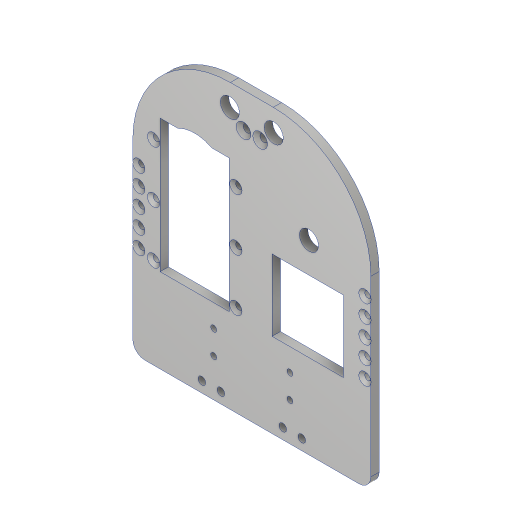
# Autodesk Inventor part: Box_Front
Saved by Autodesk Inventor 2023.2 (Build 272271000, 271)
## iProperties
Created: 2021-07-28
Part Number: Box_Front
Material: 알루미늄 6061
Document SubType Name: Modeling
Designer: user
Density: 2.7 g/cm^3
Appearance: 알루미늄 - 평지
Mass: 39.6776 g
Surface Area: 168.104 cm^2
Volume: 24.402 cm^3
Author: user
Autodesk Inventor part; units mm, degrees
ref_plane "YZ Plane" through (0, 0, 0) normal (1, 0, 0) x (0, 1, 0)
ref_plane "XZ Plane" through (0, 0, 0) normal (0, 1, 0) x (-1, 0, 0)
ref_plane "XY Plane" through (0, 0, 0) normal (0, 0, 1) x (1, 0, 0)
sketch "스케치1" plane through (0, 0, 0) normal (0, 0, 1) x (1, 0, 0)
  line L0 (-50.01, 54) -> (50.01, 54)
  line L1 (50.01, 54) -> (50.01, -40)
  line L2 (50.01, -40) -> (-50.01, -40)
  line L3 (-50.01, -40) -> (-50.01, 54)
  point P0 (0, 0)
  dimension "d0" = 100.02
  dimension "d1" = 50.01
  dimension "d2" = 94
  dimension "d40" = 40
  constraints: 8 end point, 2 parallel, 1 horizontal, 1 perpendicular
  measures "d0" distance of L1.end L2.end
  measures "d1" distance from line of L3 point (0, 0)
  measures "d2" distance between parallel lines of L2 L0
  measures "d40" distance from line of point (0, 0) L2
extrude "돌출1" add sketch "스케치1" along normal blind 3.5
sketch "스케치2" plane through (0, 0, 3.5) normal (0, 0, 1) x (1, 0, 0)
  circle A0 centre (-24.01, 13.1) radius 14
  line L0 (-50.01, -40) -> (50.01, -40) projected
  point P0 (0, 0)
  dimension "d6" = 28
  dimension "d7" = 24.01
  dimension "d8" = 53.1
  constraints: 1 centre point
  measures "d6" diameter of A0
  measures "d7" horizontal distance of point (0, 0) A0.centre
  measures "d8" distance from line of L0 A0.centre
extrude "돌출2" cut sketch "스케치2" against normal up to surface (3.5 mm away)
sketch "스케치3" plane through (0, 0, 3.5) normal (0, 0, 1) x (1, 0, 0)
  line L0 (-9.49, -29.6) -> (-38.53, -29.6)
  line L1 (-38.53, -29.6) -> (-38.53, 26.3)
  line L2 (-38.53, 26.3) -> (-9.49, 26.3)
  line L3 (-9.49, 26.3) -> (-9.49, -29.6)
  line L4 (-50.01, -40) -> (50.01, -40) projected
  circle A0 centre (-24.01, 13.1) radius 14 projected
  point P0 (0, 0)
  dimension "d11" = 10.4
  dimension "d12" = 55.9
  dimension "d13" = 29.04
  dimension "d14" = 14.52
  constraints: 8 end point, 2 parallel, 1 horizontal, 1 perpendicular
  measures "d11" distance between parallel lines of L4 L0
  measures "d12" distance between parallel lines of L0 L2
  measures "d13" distance between parallel lines of L3 L1
  measures "d14" distance from line of L1 A0.centre
extrude "돌출3" cut sketch "스케치3" against normal up to surface (3.5 mm away) contours L0 L1 L2 A0 L3 | A0 L2 picked at (-19.646, 17.031)
sketch "스케치4" plane through (0, 0, 3.5) normal (0, 0, 1) x (1, 0, 0)
  line L0 (-38.53, -29.6) -> (-38.53, 26.3) projected
  line L1 (-9.49, 26.3) -> (-9.49, -29.6) projected
  line L2 (-9.49, -29.6) -> (-38.53, -29.6) projected
  arc A0 (-19.3452, 26.3) -> (-28.6748, 26.3) centre (-24.01, 13.1) ccw projected
  arc A1 (-16.8854, 26.3) -> (-31.1346, 26.3) centre (-24.01, 13.1) ccw
  line L3 (-38.53, 26.3) -> (-28.6748, 26.3) projected
  line L4 (-19.3452, 26.3) -> (-9.49, 26.3) projected
  point P0 (0, 0)
  constraints: 2 point on circle, 2 point on line, 1 centre point, 1 coincident
extrude "돌출4" cut sketch "스케치4" against normal up to surface (3.5 mm away)
sketch "스케치5" plane through (0, 0, 3.5) normal (0, 0, 1) x (1, 0, 0)
  arc A0 (-16.8854, 26.3) -> (-31.1346, 26.3) centre (-24.01, 13.1) ccw projected
  circle A1 centre (-24.01, 13.1) radius 5
  circle A2 centre (-6.71, -4.9) radius 1.705
  circle A3 centre (-6.71, 17.1) radius 1.705
  circle A4 centre (-6.71, -26.9) radius 1.7
  circle A5 centre (-13.01, -32.2) radius 1.705
  circle A6 centre (-35.01, -32.2) radius 1.705
  circle A7 centre (-41.31, -26.9) radius 1.705
  circle A8 centre (-41.31, -4.9) radius 1.705
  circle A9 centre (-41.31, 17.1) radius 1.705
  circle A10 centre (-41.31, 17.1) radius 1.35
  circle A11 centre (-41.31, -4.9) radius 1.35
  circle A12 centre (-41.31, -26.9) radius 1.35
  circle A13 centre (-35.01, -32.2) radius 1.35
  circle A14 centre (-13.01, -32.2) radius 1.35
  circle A15 centre (-6.71, -26.9) radius 1.35
  circle A16 centre (-6.71, -4.9) radius 1.35
  circle A17 centre (-6.71, 17.1) radius 1.35
  point P0 (0, 0)
  dimension "d20" = 3.41
  dimension "d21" = 2.7
  dimension "d22" = 2.7
  dimension "d23" = 2.7
  dimension "d24" = 2.7
  dimension "d25" = 2.7
  dimension "d26" = 2.7
  dimension "d27" = 2.7
  dimension "d28" = 2.7
  constraints: 17 centre point, 8 coincident
  measures "d20" diameter of A9
  measures "d21" diameter of A10
  measures "d22" diameter of A11
  measures "d23" diameter of A12
  measures "d24" diameter of A13
  measures "d25" diameter of A14
  measures "d26" diameter of A15
  measures "d27" diameter of A16
  measures "d28" diameter of A17
extrude "돌출5" cut sketch "스케치5" against normal up to surface (3.5 mm away) contours A10 | A11 | A12 | A15 | A16 | A17
sketch "스케치6" plane through (0, 0, 3.5) normal (0, 0, 1) x (1, 0, 0)
  arc A0 (-16.8854, 26.3) -> (-31.1346, 26.3) centre (-24.01, 13.1) ccw projected
  line L0 (-24.01, 13.1) -> (24.01, 13.1)
  line L1 (-24.01, 13.1) -> (24.01, 13.1) construction
  circle A1 centre (24.01, 13.1) radius 4.025
  point P0 (0, 0)
  dimension "d31" = 48.02
  dimension "d32" = 0
  dimension "d33" = 8.05
  constraints: 4 end point, 2 horizontal, 1 centre point, 1 coincident, 1 collinear
  measures "d31" distance of L0.start L0.end
  measures "d32" distance between parallel lines of L0 L1
  measures "d33" diameter of A1
extrude "돌출6" cut sketch "스케치6" against normal up to surface (3.5 mm away)
chamfer "모따기1" distance 1.25 angle 45 6 edges at (-42.66, 17.1, 3.5) (-42.66, -4.9, 3.5) (-42.66, -26.9, 3.5) (-8.06, -26.9, 3.5) (-8.06, -4.9, 3.5) (-8.06, 17.1, 3.5)
sketch "스케치7" plane through (0, 0, 3.5) normal (0, 0, 1) x (1, 0, 0)
  circle A0 centre (24.01, 13.1) radius 4.025 projected
  arc A1 (-16.8854, 26.3) -> (-31.1346, 26.3) centre (-24.01, 13.1) ccw projected
  line L0 (24.01, 13.1) -> (9.2184, 44.8208)
  line L1 (24.01, 13.1) -> (59.01, 13.1) construction
  line L2 (-24.01, 13.1) -> (-9.2184, 44.8208)
  line L3 (-24.01, 13.1) -> (10.99, 13.1) construction
  circle A2 centre (9.2184, 44.8208) radius 4.025
  circle A3 centre (-9.2184, 44.8208) radius 4.025
  point P0 (0, 0)
  dimension "d41" = 35
  dimension "d42" = 115
  dimension "d43" = 35
  dimension "d44" = 65
  dimension "d45" = 8.05
  dimension "d46" = 8.05
  constraints: 8 end point, 2 centre point, 2 coincident, 2 equal length, 2 horizontal
  measures "d41" distance of L0.start L0.end
  measures "d42" angle of L1 L0
  measures "d43" distance of L2.start L2.end
  measures "d44" angle of L3 L2
  measures "d45" diameter of A2
  measures "d46" diameter of A3
extrude "돌출7" cut sketch "스케치7" against normal up to surface (3.5 mm away) contours A2 | A3
fillet "모깎기1" radius 41 2 edges at (50.01, 54, 1.75) (-50.01, 54, 1.75)
sketch "스케치8" plane through (0, 0, 3.5) normal (0, 0, 1) x (1, 0, 0)
  circle A0 centre (47.51, -25.5) radius 1.35
  circle A1 centre (47.51, 4.5) radius 1.35
  circle A2 centre (47.51, -18) radius 1.35
  circle A3 centre (47.51, -10.5) radius 1.35
  circle A4 centre (47.51, -3) radius 1.35
  line L0 (50.01, -40) -> (50.01, 13) projected
  line L1 (-50.01, -40) -> (50.01, -40) projected
  point P0 (0, 0)
  dimension "d50" = 2.7
  dimension "d51" = 2.7
  dimension "d52" = 2.7
  dimension "d53" = 2.7
  dimension "d54" = 2.7
  dimension "d55" = 2.5
  dimension "d56" = 2.5
  dimension "d57" = 2.5
  dimension "d58" = 2.5
  dimension "d59" = 2.5
  dimension "d60" = 14.5
  dimension "d61" = 44.5
  dimension "d62" = 22
  dimension "d63" = 29.5
  dimension "d64" = 37
  constraints: 5 centre point
  measures "d50" diameter of A0
  measures "d51" diameter of A1
  measures "d52" diameter of A2
  measures "d53" diameter of A3
  measures "d54" diameter of A4
  measures "d55" distance from line of L0 A0.centre
  measures "d56" distance from line of L0 A1.centre
  measures "d57" distance from line of L0 A2.centre
  measures "d58" distance from line of L0 A3.centre
  measures "d59" distance from line of L0 A4.centre
  measures "d60" distance from line of L1 A0.centre
  measures "d61" distance from line of L1 A1.centre
  measures "d62" distance from line of L1 A2.centre
  measures "d63" distance from line of L1 A3.centre
  measures "d64" distance from line of L1 A4.centre
extrude "돌출8" cut sketch "스케치8" against normal up to surface (3.5 mm away)
chamfer "모따기2" distance 1.25 angle 45 5 edges at (46.16, -25.5, 3.5) (46.16, -18, 3.5) (46.16, -10.5, 3.5) (46.16, -3, 3.5) (46.16, 4.5, 3.5)
sketch "스케치9" plane through (0, 0, 3.5) normal (0, 0, 1) x (1, 0, 0)
  line L0 (0, 0) -> (0, -40)
  line L1 (-50.01, -40) -> (50.01, -40) projected
  circle A0 centre (47.51, 4.5) radius 1.35 projected
  circle A1 centre (47.51, -3) radius 1.35 projected
  circle A2 centre (47.51, -10.5) radius 1.35 projected
  circle A3 centre (47.51, -18) radius 1.35 projected
  circle A4 centre (47.51, -25.5) radius 1.35 projected
  circle A5 centre (-47.51, 4.5) radius 1.35
  circle A6 centre (-47.51, -3) radius 1.35
  circle A7 centre (-47.51, -10.5) radius 1.35
  circle A8 centre (-47.51, -18) radius 1.35
  circle A9 centre (-47.51, -25.5) radius 1.35
  constraints: 5 centre point, 5 symmetric about line, 2 end point, 1 midpoint, 5 other
extrude "돌출9" cut sketch "스케치9" against normal up to surface (3.5 mm away) contours A5 | A6 | A7 | A8 | A9
chamfer "모따기3" distance 1.25 angle 45 5 edges at (-48.86, 4.5, 3.5) (-48.86, -3, 3.5) (-48.86, -10.5, 3.5) (-48.86, -18, 3.5) (-48.86, -25.5, 3.5)
sketch "스케치10" plane through (0, 0, 3.5) normal (0, 0, 1) x (1, 0, 0)
  line L0 (-50.01, -26.2141) -> (-50.01, -40) projected
  line L1 (-50.01, -40) -> (50.01, -40) projected
  line L2 (50.01, -40) -> (50.01, -26.2141) projected
  line L3 (-50.01, -40) -> (50.01, -40)
  line L4 (50.01, -40) -> (50.01, -65)
  line L5 (50.01, -65) -> (-50.01, -65)
  line L6 (-50.01, -65) -> (-50.01, -40)
  point P0 (0, 0)
  dimension "d75" = 25
  dimension "d76" = 100.02
  constraints: 8 end point, 2 parallel, 1 horizontal, 1 perpendicular
  measures "d75" distance of L3.end L4.end
  measures "d76" distance between parallel lines of L4 L6
extrude "돌출10" add sketch "스케치10" against normal up to surface (3.5 mm away)
sketch "스케치11" plane through (0, 0, 3.5) normal (0, 0, 1) x (1, 0, 0)
  line L0 (-25, -58) -> (25, -58)
  line L1 (25, -58) -> (25, -63)
  line L2 (25, -63) -> (-25, -63)
  line L3 (-25, -63) -> (-25, -58)
  line L4 (50.01, -65) -> (-50.01, -65) projected
  circle A0 centre (-21, -60.5) radius 1.6
  circle A1 centre (-13, -60.5) radius 1.6
  circle A2 centre (13, -60.5) radius 1.6
  circle A3 centre (21, -60.5) radius 1.6
  point P0 (0, 0)
  dimension "d79" = 50
  dimension "d80" = 5
  dimension "d81" = 25
  dimension "d82" = 7
  dimension "d83" = 3.2
  dimension "d84" = 3.2
  dimension "d85" = 3.2
  dimension "d86" = 3.2
  dimension "d87" = 4
  dimension "d88" = 2.5
  dimension "d89" = 2.5
  dimension "d90" = 12
  dimension "d91" = 2.5
  dimension "d92" = 2.5
  dimension "d93" = 4
  dimension "d94" = 12
  constraints: 8 end point, 4 centre point, 2 parallel, 1 horizontal, 1 perpendicular
  measures "d79" distance of L1.end L2.end
  measures "d80" distance of L0.end L1.end
  measures "d81" distance from line of L1 point (0, 0)
  measures "d82" distance between parallel lines of L4 L0
  measures "d83" diameter of A0
  measures "d84" diameter of A1
  measures "d85" diameter of A2
  measures "d86" diameter of A3
  measures "d87" distance from line of L3 A0.centre
  measures "d88" distance from line of L2 A1.centre
  measures "d89" distance from line of L2 A0.centre
  measures "d90" distance from line of A1.centre L3
  measures "d91" distance from line of L2 A2.centre
  measures "d92" distance from line of L2 A3.centre
  measures "d93" distance from line of L1 A3.centre
  measures "d94" distance from line of L1 A2.centre
extrude "돌출11" cut sketch "스케치11" against normal up to surface (3.5 mm away) contours A0 | A1 | A2 | A3
fillet "모깎기2" radius 5 2 edges at (50.01, -65, 1.75) (-50.01, -65, 1.75)
sketch "스케치13" plane through (0, 0, 0) normal (0, 0, -1) x (-1, 0, 0)
  line L0 (9.49, 26.3) -> (16.8854, 26.3) projected
  line L1 (7, 36.3) -> (-7, 36.3)
  line L2 (-7, 36.3) -> (-7, 42.3)
  line L3 (-7, 42.3) -> (7, 42.3)
  line L4 (7, 42.3) -> (7, 36.3)
  circle A0 centre (3.5, 39.3) radius 1.6
  circle A1 centre (-3.5, 39.3) radius 1.6
  point P0 (0, 0)
  dimension "d124" = 14
  dimension "d125" = 6
  dimension "d126" = 7
  dimension "d127" = 16
  dimension "d128" = 3.2
  dimension "d129" = 3.2
  dimension "d130" = 3.5
  dimension "d131" = 3.5
  dimension "d132" = 3
  dimension "d133" = 3
  constraints: 8 end point, 2 centre point, 2 parallel, 1 horizontal, 1 perpendicular
  measures "d124" distance of L2.end L3.end
  measures "d125" distance of L1.end L2.end
  measures "d126" distance from line of point (0, 0) L2
  measures "d127" distance between parallel lines of L3 L0
  measures "d128" diameter of A0
  measures "d129" diameter of A1
  measures "d130" distance from line of L4 A0.centre
  measures "d131" distance from line of L2 A1.centre
  measures "d132" distance from line of L3 A0.centre
  measures "d133" distance from line of L3 A1.centre
extrude "돌출13" cut sketch "스케치13" against normal up to surface (3.5 mm away) contours A0 | A1
chamfer "모따기5" distance 1.5 angle 45 2 edges at (5.1, 39.3, 3.5) (-1.9, 39.3, 3.5)
sketch "스케치17" plane through (0, 0, 3.5) normal (0, 0, 1) x (1, 0, 0)
  line L0 (-20, -31.5) -> (20, -31.5)
  line L1 (20, -31.5) -> (20, -56.5)
  line L2 (20, -56.5) -> (-20, -56.5)
  line L3 (-20, -56.5) -> (-20, -31.5)
  line L4 (-20, -31.5) -> (20, -56.5) construction
  line L5 (20, -31.5) -> (-20, -56.5) construction
  line L6 (45.01, -65) -> (-45.01, -65) projected
  point P0 (0, 0)
  point P1 (0, -44)
  point P2 (0, -65)
  dimension "d150" = 40
  dimension "d151" = 25
  dimension "d152" = 21
  constraints: 12 end point, 3 midpoint, 2 parallel, 1 horizontal, 1 perpendicular, 1 vertical alignment
  measures "d150" distance of L1.end L2.end
  measures "d151" distance of L0.end L1.end
  measures "d152" distance of point (0, -44) point (0, -65)
extrude "돌출17" add sketch "스케치17" along normal blind 26
sketch "스케치19" plane through (0, 0, 29.5) normal (0, 0, 1) x (1, 0, 0)
  line L0 (-20, -56.5) -> (20, -56.5) projected
  line L1 (20, -56.5) -> (20, -31.5) projected
  line L2 (20, -31.5) -> (-20, -31.5) projected
  line L3 (-20, -31.5) -> (-20, -56.5) projected
  circle A0 centre (-16, -39) radius 1.25
  circle A1 centre (-16, -49) radius 1.25
  line L4 (20, -31.5) -> (-20, -31.5) projected
  line L5 (0, -31.5) -> (0, -56.5)
  circle A2 centre (16, -39) radius 1.25
  circle A3 centre (16, -49) radius 1.25
  point P0 (0, 0)
  dimension "d155" = 10
  dimension "d156" = 2.5
  dimension "d157" = 4
  dimension "d158" = 7.5
  constraints: 4 centre point, 2 end point, 2 midpoint, 2 symmetric about line, 1 equal radius, 1 vertical alignment, 2 other
  measures "d155" distance of A0.centre A1.centre
  measures "d156" diameter of A0
  measures "d157" distance from line of L3 A0.centre
  measures "d158" distance from line of L0 A1.centre
extrude "돌출18" cut sketch "스케치19" against normal blind 26 contours A0 | A1 | A2 | A3
sketch "스케치20" plane through (0, 0, 29.5) normal (0, 0, 1) x (1, 0, 0)
  circle A0 centre (16, -39) radius 1.25 projected
  circle A1 centre (-16, -49) radius 1.25 projected
  circle A2 centre (16, -49) radius 1.25 projected
  circle A3 centre (-16, -39) radius 1.25 projected
  line L0 (-20, -56.5) -> (20, -56.5) projected
  line L1 (20, -56.5) -> (20, -31.5) projected
  line L2 (20, -31.5) -> (-20, -31.5) projected
  line L3 (-20, -31.5) -> (-20, -56.5) projected
  line L4 (-6, -36.5) -> (6, -36.5)
  line L5 (10, -40.5) -> (10, -47.5)
  line L6 (6, -51.5) -> (-6, -51.5)
  line L7 (-10, -47.5) -> (-10, -40.5)
  line L8 (-10, -36.5) -> (10, -51.5) construction
  line L9 (10, -36.5) -> (-10, -51.5) construction
  line L10 (-20, -56.5) -> (20, -56.5) projected
  arc A4 (-6, -36.5) -> (-10, -40.5) centre (-6, -40.5) ccw
  arc A5 (10, -40.5) -> (6, -36.5) centre (6, -40.5) ccw
  arc A6 (6, -51.5) -> (10, -47.5) centre (6, -47.5) ccw
  arc A7 (-10, -47.5) -> (-6, -51.5) centre (-6, -47.5) ccw
  point P0 (0, 0)
  point P1 (0, -44)
  point P2 (0, -56.5)
  point P3 (0, -56.5)
  point P4 (0, -51.5)
  dimension "d161" = 20
  dimension "d162" = 15
  dimension "d164" = 5
  dimension "d165" = 4
  constraints: 12 end point, 8 point on circle, 8 point on line, 8 tangent, 5 midpoint, 4 centre point, 3 equal radius, 2 parallel, 1 horizontal, 1 perpendicular
  measures "d161" distance of L8.end L9.end
  measures "d162" distance of L9.start L8.end
  measures "d164" distance of point (0, -56.5) point (0, -51.5)
  measures "d165" radius of A4
extrude "돌출19" cut sketch "스케치20" against normal blind 26 contours L4 A5 L5 A6 L6 A7 L7 A4
fillet "모깎기3" radius 4 4 edges at (-20, -31.5, 16.5) (-20, -56.5, 16.5) (20, -56.5, 16.5) (20, -31.5, 16.5)
sketch "스케치21" plane through (0, 0, 29.5) normal (0, 0, 1) x (1, 0, 0)
  arc A0 (6, -51.5) -> (10, -47.5) centre (6, -47.5) ccw projected
  line L0 (6, -51.5) -> (-6, -51.5) projected
  arc A1 (-10, -47.5) -> (-6, -51.5) centre (-6, -47.5) ccw projected
  line L1 (-10, -47.5) -> (-10, -40.5) projected
  arc A2 (-6, -36.5) -> (-10, -40.5) centre (-6, -40.5) ccw projected
  line L2 (-6, -36.5) -> (6, -36.5) projected
  arc A3 (10, -40.5) -> (6, -36.5) centre (6, -40.5) ccw projected
  line L3 (10, -40.5) -> (10, -47.5) projected
  circle A4 centre (16, -39) radius 1.25 projected
  circle A5 centre (-16, -49) radius 1.25 projected
  circle A6 centre (16, -49) radius 1.25 projected
  circle A7 centre (-16, -39) radius 1.25 projected
  arc A8 (20, -35.5) -> (16, -31.5) centre (16, -35.5) ccw projected
  line L4 (16, -31.5) -> (-16, -31.5) projected
  arc A9 (-16, -31.5) -> (-20, -35.5) centre (-16, -35.5) ccw projected
  line L5 (-20, -35.5) -> (-20, -52.5) projected
  arc A10 (-20, -52.5) -> (-16, -56.5) centre (-16, -52.5) ccw projected
  line L6 (-16, -56.5) -> (16, -56.5) projected
  arc A11 (16, -56.5) -> (20, -52.5) centre (16, -52.5) ccw projected
  line L7 (20, -52.5) -> (20, -35.5) projected
  point P0 (0, 0)
extrude "돌출20" cut sketch "스케치21" against normal up to surface (29.5 mm away) contours A4 | A5 | A6 | A7
sketch "스케치22" plane through (0, 0, 29.5) normal (0, 0, 1) x (1, 0, 0)
  arc A0 (6, -51.5) -> (10, -47.5) centre (6, -47.5) ccw projected
  line L0 (6, -51.5) -> (-6, -51.5) projected
  arc A1 (-10, -47.5) -> (-6, -51.5) centre (-6, -47.5) ccw projected
  line L1 (-10, -47.5) -> (-10, -40.5) projected
  arc A2 (-6, -36.5) -> (-10, -40.5) centre (-6, -40.5) ccw projected
  line L2 (-6, -36.5) -> (6, -36.5) projected
  arc A3 (10, -40.5) -> (6, -36.5) centre (6, -40.5) ccw projected
  line L3 (10, -40.5) -> (10, -47.5) projected
  circle A4 centre (16, -39) radius 1.25 projected
  circle A5 centre (-16, -49) radius 1.25 projected
  circle A6 centre (16, -49) radius 1.25 projected
  circle A7 centre (-16, -39) radius 1.25 projected
  arc A8 (20, -35.5) -> (16, -31.5) centre (16, -35.5) ccw projected
  line L4 (16, -31.5) -> (-16, -31.5) projected
  arc A9 (-16, -31.5) -> (-20, -35.5) centre (-16, -35.5) ccw projected
  line L5 (-20, -35.5) -> (-20, -52.5) projected
  arc A10 (-20, -52.5) -> (-16, -56.5) centre (-16, -52.5) ccw projected
  line L6 (-16, -56.5) -> (16, -56.5) projected
  arc A11 (16, -56.5) -> (20, -52.5) centre (16, -52.5) ccw projected
  line L7 (20, -52.5) -> (20, -35.5) projected
  point P0 (0, 0)
extrude "돌출21" cut sketch "스케치22" against normal up to surface (26 mm away)
sketch "스케치23" plane through (0, 0, 3.5) normal (0, 0, 1) x (1, 0, 0)
  line L0 (8.51, -29.6) -> (38.51, -29.6)
  line L1 (38.51, -29.6) -> (38.51, 0.4)
  line L2 (38.51, 0.4) -> (8.51, 0.4)
  line L3 (8.51, 0.4) -> (8.51, -29.6)
  line L4 (8.51, -29.6) -> (38.51, 0.4) construction
  line L5 (38.51, -29.6) -> (8.51, 0.4) construction
  line L6 (45.01, -65) -> (-45.01, -65) projected
  line L7 (50.01, -26.2141) -> (50.01, -60) projected
  point P0 (0, 0)
  point P1 (23.51, -14.6)
  dimension "d173" = 30
  dimension "d174" = 30
  dimension "d175" = 35.4
  dimension "d176" = 11.5
  constraints: 12 end point, 2 midpoint, 2 parallel, 1 horizontal, 1 perpendicular
  measures "d173" distance of L2.end L1.end
  measures "d174" distance of L1.end L0.end
  measures "d175" distance between parallel lines of L6 L0
  measures "d176" distance between parallel lines of L7 L1
extrude "돌출22" cut sketch "스케치23" against normal blind 10
sketch "스케치15" plane through (0, 0, 3.5) normal (0, 0, 1) x (1, 0, 0)
  circle A0 centre (24.01, 13.1) radius 4.025 projected
  circle A1 centre (24.01, 13.1) radius 4.8
  point P0 (0, 0)
  dimension "d143" = 9.6
  constraints: 1 centre point, 1 coincident
  measures "d143" diameter of A1
equation "\"d1\" = 0.5 * d0"
equation "\"d14\" = 0.5 * d13"
equation "\"d81\" = 0.5 * d79"
equation "\"d126\" = 0.5 * d124"
